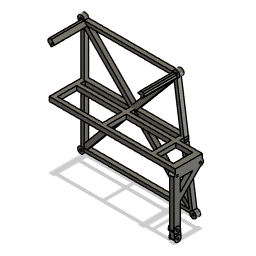
ITX_1 (Autodesk Fusion 360 design; units mm, degrees)
Autodesk Fusion 360 part; units mm, degrees
note: some values were not read from the file. Set by a fixed rule: which face or edge a step refers to.
sketch "草图1" plane through (0, 0, 0) normal (0, 1, 0) x (1, 0, 0)
  line L0 (0, 0) -> (81.5, 0)
  line L1 (81.5, 0) -> (81.5, -40.5)
  line L2 (81.5, -40.5) -> (0, -40.5)
  line L3 (0, -40.5) -> (0, 0)
  line L4 (81.5, -40.5) -> (-5, -40.5)
  line L5 (-5, -40.5) -> (-5, 5)
  line L6 (-5, 5) -> (81.5, 5)
  line L7 (81.5, 5) -> (81.5, -40.5)
  line L8 (0, 0) -> (86.5, 0)
  line L9 (86.5, 0) -> (86.5, -45.5)
  line L10 (86.5, -45.5) -> (0, -45.5)
  line L11 (0, -45.5) -> (0, 0)
  line L12 (-5, 5) -> (86.5, 5)
  line L13 (86.5, 5) -> (86.5, -45.5)
  line L14 (86.5, -45.5) -> (-5, -45.5)
  line L15 (-5, -45.5) -> (-5, 5)
  line L16 (-6, 6) -> (87.5, 6)
  line L17 (87.5, 6) -> (87.5, -46.5)
  line L18 (87.5, -46.5) -> (-6, -46.5)
  line L19 (-6, -46.5) -> (-6, 6)
  line L20 (-1, -41.5) -> (82.5, -41.5)
  line L21 (82.5, -41.5) -> (82.5, 1)
  line L22 (82.5, 1) -> (-1, 1)
  line L23 (-1, 1) -> (-1, -41.5)
  dimension "d1" = 81.5
  dimension "d2" = 40.5
  dimension "d3" = 5
  dimension "d4" = 5
  dimension "d5" = 5
  dimension "d6" = 5
  dimension "d7" = 1
  dimension "d8" = 1
  dimension "d9" = 1
  dimension "d10" = 1
  dimension "d11" = 1
  dimension "d12" = 1
  dimension "d13" = 1
  dimension "d14" = 1
  dimension "d15" = 4
  constraint horizontal L0
  constraint vertical L1
  constraint horizontal L2
  constraint vertical L3
  constraint coincident L0.start L3.end
  constraint horizontal L4
  constraint vertical L5
  constraint horizontal L6
  constraint vertical L7
  constraint horizontal L8
  constraint vertical L9
  constraint horizontal L10
  constraint vertical L11
  constraint horizontal L12
  constraint vertical L13
  constraint horizontal L14
  constraint vertical L15
  constraint horizontal L16
  constraint vertical L17
  constraint horizontal L18
  constraint vertical L19
  constraint horizontal L20
  constraint vertical L21
  constraint horizontal L22
  constraint vertical L23
  measures "d1" distance of L0.start L0.end
  measures "d2" distance of L0.start L2.end
  measures "d3" distance of L3 L5
  measures "d4" distance of L0 L6
  measures "d5" distance of L1 L9
  measures "d6" distance of L4 L10
  measures "d7" distance of L12 L16
  measures "d8" distance of L5 L19
  measures "d9" distance of L10 L18
  measures "d10" distance of L9 L17
  measures "d11" distance of L8 L22
  measures "d12" distance of L3 L23
  measures "d13" distance of L2 L20
  measures "d14" distance of L7 L21
  measures "d15" distance of L9 L21
extrude "拉伸1" add sketch "草图1" along normal blind 160 contours L4 L5 L6 L7 L12 L15 L22 L23 | L7 L8 L12 L13 L21 L22 | L8 L9 L10 L11 L13 L14 L20 L21 | L4 L11 L14 L15 L20 L23 makes body 1
extrude "拉伸2" add sketch "草图1" against normal blind 4 separate body contours L4 L5 L6 L7 L12 L15 L22 L23 | L7 L8 L12 L13 L21 L22 | L8 L9 L10 L11 L13 L14 L20 L21 | L4 L11 L14 L15 L20 L23 makes body 2
extrude "拉伸3" add 2 faces at (54, -1.3333, -1) (82.1667, -1.3333, -1) along direction (0, 0, 1) blind 42.5 separate body on bodies 2 makes body 3
sketch "草图2" plane through (0, 0, -5) normal (0, 0, -1) x (-1, 0, 0)
  line L0 (-86.5, 0) -> (5, 0)
  line L1 (5, 0) -> (5, 160)
  line L2 (5, 160) -> (-86.5, 160)
  line L3 (-86.5, 160) -> (-86.5, 0)
  line L4 (5, 160) -> (-165, 160)
  line L5 (-165, 160) -> (-165, -10)
  line L6 (-165, -10) -> (5, -10)
  line L7 (5, -10) -> (5, 160)
  line L8 (5, 160) -> (-166, 160)
  line L9 (-166, 160) -> (-166, -11)
  line L10 (-166, -11) -> (5, -11)
  line L11 (5, -11) -> (5, 160)
  line L12 (-166, -11) -> (6, -11)
  line L13 (6, -11) -> (6, 161)
  line L14 (6, 161) -> (-166, 161)
  line L15 (-166, 161) -> (-166, -11)
  circle A0 centre (-131.98, 153.83) radius 1.5
  circle A1 centre (0.1, 153.83) radius 1.5
  circle A2 centre (-154.84, -3.65) radius 1.5
  circle A3 centre (0.1, -3.65) radius 1.5
  line L16 (-131.98, 153.83) -> (0.1, 153.83)
  line L17 (-154.84, -3.65) -> (0.1, -3.65)
  circle A4 centre (-131.98, 153.83) radius 4.5
  circle A5 centre (0.1, 153.83) radius 4.5
  circle A6 centre (0.1, -3.65) radius 4.5
  circle A7 centre (-154.84, -3.65) radius 4.5
  line L18 (-131.98, 153.83) -> (-154.84, -3.65)
  line L19 (0.1, 153.83) -> (0.1, -3.65)
  line L20 (-127.48, 153.83) -> (-150.34, -3.65)
  line L21 (-4.4, 153.83) -> (-4.4, -3.65)
  line L22 (0.1, 153.83) -> (4.6, 153.83)
  line L23 (0.1, -3.65) -> (4.6, -3.65)
  line L24 (4.6, -3.65) -> (4.6, 153.83)
  line L25 (-132.6265, 149.3767) -> (-131.3335, 158.2833)
  line L26 (-131.3335, 158.2833) -> (0.0984, 158.33)
  line L27 (-154.1935, 0.8033) -> (-155.4865, -8.1033)
  line L28 (-155.4865, -8.1033) -> (0.0986, -8.15)
  line L29 (-154.1935, 0.8033) -> (0.1, 0.85)
  line L30 (-132.6265, 149.3767) -> (0.1, 149.33)
  line L31 (-132.6265, 149.3767) -> (-4.4, -3.65)
  line L32 (0.1, 0.85) -> (-127.48, 153.83)
  line L33 (-154.1935, 0.8033) -> (-4.4, 153.83)
  line L34 (0.1, 149.33) -> (-150.34, -3.65)
  line L35 (-165, 160) -> (-165, 1)
  dimension "d22" = 170
  dimension "d23" = 170
  dimension "d24" = 1
  dimension "d25" = 1
  dimension "d26" = 1
  dimension "d27" = 1
  dimension "d28" = 3
  dimension "d29" = 3
  dimension "d30" = 3
  dimension "d31" = 3
  dimension "d32" = 132.08
  dimension "d33" = 157.48
  dimension "d34" = 157.48
  dimension "d35" = 154.94
  dimension "d36" = 6.35
  dimension "d37" = 22.86
  dimension "d38" = 10.16
  dimension "d39" = 9
  dimension "d40" = 9
  dimension "d41" = 9
  dimension "d42" = 9
  dimension "d84" = 159
  constraint horizontal L4
  constraint vertical L5
  constraint horizontal L6
  constraint vertical L7
  constraint coincident L1.end L2.start
  constraint horizontal L8
  constraint vertical L9
  constraint horizontal L10
  constraint vertical L11
  constraint horizontal L12
  constraint vertical L13
  constraint horizontal L14
  constraint vertical L15
  constraint coincident A0.centre L16.start
  constraint coincident A1.centre L16.end
  constraint coincident A2.centre L17.start
  constraint coincident A3.centre L17.end
  constraint concentric A2 A7
  constraint coincident A4 L20.start
  constraint coincident L16 L20.start
  constraint coincident A7 L20.end
  constraint coincident L17 L20.end
  constraint coincident A5 L21.start
  constraint coincident L16 L21.start
  constraint coincident L17 L21.end
  constraint coincident A6 L21.end
  constraint tangent A6 L21
  constraint coincident A5 L22.end
  constraint perpendicular L7 L22
  constraint coincident A6 L23.end
  constraint perpendicular L7 L23
  constraint coincident A4 L25.start
  constraint coincident L18 L25.start
  constraint coincident A4 L25.end
  constraint parallel L18 L25
  constraint coincident A5 L26.end
  constraint tangent A5 L26
  constraint coincident A7 L27.start
  constraint coincident L18 L27.start
  constraint coincident A7 L27.end
  constraint parallel L18 L27
  constraint coincident A6 L28.end
  constraint tangent A6 L28
  constraint coincident A6 L29.end
  constraint coincident L19 L29.end
  constraint coincident A5 L30.end
  constraint coincident L19 L30.end
  constraint perpendicular L4 L35
  measures "d22" distance of L1.end L4.end
  measures "d23" distance of L1.end L6.end
  measures "d24" distance of L5 L9
  measures "d25" distance of L6 L10
  measures "d26" distance of L4 L14
  measures "d27" distance of L11 L13
  measures "d28" diameter of A0
  measures "d29" diameter of A1
  measures "d30" diameter of A2
  measures "d31" diameter of A3
  measures "d32" horizontal distance of A0.centre A1.centre
  measures "d33" vertical distance of A0.centre A2.centre
  measures "d34" vertical distance of A1.centre A3.centre
  measures "d35" horizontal distance of A2.centre A3.centre
  measures "d36" distance of L6 A2.centre
  measures "d37" horizontal distance of A0.centre A2.centre
  measures "d38" distance of L5 A2.centre
  measures "d39" diameter of A4
  measures "d40" diameter of A5
  measures "d41" diameter of A6
  measures "d42" diameter of A7
  measures "d84" distance of L4.end L35.end
extrude "拉伸4" add sketch "草图2" along normal blind 6 separate body contours L0 A6 L19 | L0 A3 L17 A6 L19 | A3 L17 A6 L23 | L0 A6 L19 | A2 L17 A7 L27 L28 | A2 L17 A7 L18 L27 | L0 A3 A6 L19 L23 | A2 A7 L18 L27 | A7 L28 | A1 A5 L19 L22 | A1 L16 A5 L19 | A4 L30 | A0 A4 L18 L25 | A0 L16 A4 L18 L20 L25 L30 | A1 L16 A5 L22 | A0 L16 A4 L25 | A4 L20 makes body 4 at (-4.2466, 152.082, -9) makes body 5 at (-4.5776, -4.0981, -7) makes body 6 at (127.4856, 154.0543, -7) makes body 7 at (150.3624, -3.2019, -9)
extrude "拉伸5" add sketch "草图2" along normal blind 6 separate body contours L0 L3 L29 L31 | L0 L3 L17 L29 L31 L34 | L0 L21 L29 L31 | L0 L21 L31 | L21 L29 L32 | L19 L21 L32 L34 | L0 A6 L21 L29 | L0 A6 L21 | L20 L29 L34 | A7 L20 L29 | L20 L29 L33 | L18 L20 L31 L33 | A5 L21 L30 | L21 L30 L34 | A4 L20 L30 L31 | L3 L16 L30 L33 | L21 L30 L33 | A4 L20 L30 | L3 L16 L30 L32 | A4 L20 L30 L32 makes body 8
extrude "拉伸6" add sketch "草图2" along normal blind 6 separate body contours L21 L29 L31 L32 L34 | L3 L20 L29 L33 L34 | L3 L31 L33 L34 | L31 L32 L33 L34 | L3 L31 L32 L33 | L21 L30 L32 L33 L34 | L3 L20 L30 L31 L32 makes body 9
move_body "移动1" bodies 1 3 2 to x (1, 0, 0) y (0, 1, 0) z (0, 0, 1) at (10, 0, 0)
move_body "移动2" bodies 1 3 2 to x (0, 1, 0) y (-1, 0, 0) z (0, 0, 1) at (92.5, -100.5, 0)
move_body "移动3" bodies 2 3 1 to x (1, 0, 0) y (0, 1, 0) z (0, 0, 1) at (69.5, 84.5, 0)
sketch "草图3" plane through (166, 0, 0) normal (1, 0, 0) x (0, 0, -1)
  line L0 (1, -7) -> (1, 76.5)
  line L1 (1, 76.5) -> (-41.5, 76.5)
  line L2 (-41.5, 76.5) -> (-41.5, -7)
  line L3 (-41.5, -7) -> (1, -7)
  circle A0 centre (-36, 73) radius 1.5
  circle A1 centre (-4, 73.0152) radius 1.5
  circle A2 centre (-35, -2.6) radius 1.5
  circle A3 centre (-36, 8.2) radius 1.5
  line L4 (-36, 8.2) -> (-36, 73)
  circle A4 centre (-35, -2.6) radius 4.4
  circle A5 centre (-36, 8.2) radius 4.4
  circle A6 centre (-36, 73) radius 4.4
  circle A7 centre (-4, 73.0152) radius 4.4
  line L5 (-33.3335, 76.5) -> (-6.6863, 76.5)
  line L6 (-36, 68.6) -> (-3.9979, 68.6152)
  line L7 (-36, 73) -> (-40.4, 73)
  line L8 (-36, 8.2) -> (-40.4, 8.2)
  line L9 (-35, -2.6) -> (-39.4, -2.6)
  line L10 (-39.4, -2.6) -> (-40.4, 8.2)
  line L11 (-40.4, 8.2) -> (-40.4, 73)
  line L12 (-36, 8.2) -> (-31.6, 8.2)
  line L13 (-31.6, 8.2) -> (-31.6, 73)
  line L14 (-36, 73) -> (-31.6, 73)
  line L15 (-35, -2.6) -> (-30.6, -2.6)
  line L16 (-31.6, 8.2) -> (-30.6, -2.6)
  line L17 (-4, 73.0152) -> (0.4, 73.0152)
  line L18 (-3.9979, 68.6152) -> (-31.6, 40.6)
  line L19 (-6.6863, 76.5) -> (-31.6, 51.2134)
  dimension "d50" = 3
  dimension "d51" = 3
  dimension "d52" = 3
  dimension "d53" = 3
  dimension "d54" = 32
  dimension "d56" = 15.2
  dimension "d57" = 4.4
  dimension "d58" = 36
  dimension "d59" = 37
  dimension "d60" = 8.8
  dimension "d61" = 8.8
  dimension "d62" = 8.8
  dimension "d63" = 8.8
  constraint coincident A3.centre L4.start
  constraint coincident A0.centre L4.end
  constraint concentric A2 A4
  constraint concentric A3 A5
  constraint concentric A0 A6
  constraint concentric A1 A7
  constraint coincident A6 L5.start
  constraint coincident L1 L5.start
  constraint coincident A7 L5.end
  constraint coincident L1 L5.end
  constraint coincident A6 L6.start
  constraint coincident L4 L6.start
  constraint coincident A7 L6.end
  constraint tangent A7 L6
  constraint coincident A6 L7.end
  constraint perpendicular L4 L7
  constraint coincident A5 L8.end
  constraint perpendicular L4 L8
  constraint coincident A2.centre A4.centre
  constraint coincident A4 L9.end
  constraint parallel L8 L9
  constraint coincident A5 L12.end
  constraint parallel L8 L12
  constraint coincident A6 L13.end
  constraint tangent A6 L13
  constraint coincident A4 L15.end
  constraint parallel L9 L15
  constraint coincident A1.centre A7.centre
  constraint coincident A7 L17.end
  constraint perpendicular L0 L17
  constraint midpoint L13 L18.end
  constraint coincident L13 L19.end
  constraint parallel L18 L19
  measures "d50" diameter of A0
  measures "d51" diameter of A1
  measures "d52" diameter of A2
  measures "d53" diameter of A3
  measures "d54" distance of A0.centre A1.centre
  measures "d56" distance of L3 A3.centre
  measures "d57" distance of L3 A2.centre
  measures "d58" distance of L0 A2.centre
  measures "d59" distance of L0 A3.centre
  measures "d60" diameter of A4
  measures "d61" diameter of A5
  measures "d62" diameter of A6
  measures "d63" diameter of A7
extrude "拉伸7" add sketch "草图3" along normal blind 8 separate body contours A2 A4 L9 L15 | L1 A7 L19 | A2 A4 L9 L15 L16 | A4 L16 | A7 L19 | A3 A5 L8 L10 L12 | A5 L10 | L1 A0 A6 L7 L14 | A3 L4 A5 L12 | A3 L4 A5 L8 | A0 L4 A6 L14 | A0 L4 A6 L7 makes body 10 at (171.3333, 72.3225, 40.3475) makes body 11 at (168.6667, -3.0381, 30.6219) makes body 12 at (171.3333, 76.2221, 7.0126) makes body 13 at (168.6667, 7.7619, 31.6219)
extrude "拉伸8" add sketch "草图3" along normal blind 8 separate body contours A4 A5 L10 L16 | L1 A6 A7 L5 L6 L13 L19 | A7 L6 L19 | L6 L13 L18 L19 | L4 A5 L6 L13 | L4 A5 A6 L11 | A6 L6 L13 makes body 14
extrude "拉伸9" add 3 faces at (168.6667, 76.5, 35.1112) (168.6667, 76.5, 15.5687) (171.3333, 76.5, 3.1046) along direction (0, 1, 0) blind 6 separate body on bodies 10 12 14 makes body 15
extrude "拉伸10" add 3 faces at (166, 80.5, 35.1112) (166, 78.5, 15.5687) (166, 78.5, 3.1046) along direction (-1, 0, 0) blind 166.1 on bodies 15 bodies 14 15 10 12
extrude "拉伸11" add 1 faces at (113.3, 80.5, 1.3137) along direction (0, 0, -1) blind 12.314 separate body on bodies 14 makes body 16
extrude "拉伸12" cut 1 faces at (174, 78.5, -2.791) along direction (-1, 0, 0) blind 31.173 on bodies 16 bodies 8 16
combine "合并1" operation add target body 14 tool bodies 16
sketch "草图4" plane through (0, 82.5, 0) normal (0, 1, 0) x (-1, 0, 0)
  line L0 (0.1, 38.6665) -> (-174, 38.6665)
  line L1 (-174, 38.6665) -> (-174, 1.3137)
  line L2 (-174, 1.3137) -> (-142.827, 1.3137)
  line L3 (-142.827, 1.3137) -> (-142.827, -11.0003)
  line L4 (-142.827, -11.0003) -> (0.1, -11.0003)
  line L5 (0.1, -11.0003) -> (0.1, 38.6665)
  line L6 (0.1, 38.6665) -> (-5.9, 38.6665)
  line L7 (-174, 38.6665) -> (-166, 38.6665)
  line L8 (-142.827, 1.3137) -> (-142.827, 38.6665)
  line L9 (-142.827, 38.6665) -> (-136.827, 38.6665)
  line L10 (-71.3635, -11.0003) -> (-71.3635, 38.6665)
  line L11 (-71.3635, 38.6665) -> (-68.3635, 38.6665)
  line L12 (-71.3635, 38.6665) -> (-74.3635, 38.6665)
  line L13 (-5.9, 38.6665) -> (-68.3635, 38.6665)
  line L14 (-68.3635, 38.6665) -> (-68.3635, -11.0003)
  line L15 (-68.3635, -11.0003) -> (-5.9, -11.0003)
  line L16 (-5.9, -11.0003) -> (-5.9, 38.6665)
  line L17 (-74.3635, 38.6665) -> (-136.827, 38.6665)
  line L18 (-136.827, 38.6665) -> (-136.827, -11.0003)
  line L19 (-136.827, -11.0003) -> (-74.3635, -11.0003)
  line L20 (-74.3635, -11.0003) -> (-74.3635, 38.6665)
  line L21 (-5.9, 38.6665) -> (-142.827, 38.6665)
  line L22 (-142.827, 38.6665) -> (-142.827, -4.8433)
  line L23 (-142.827, -4.8433) -> (-5.9, -4.8433)
  line L24 (-5.9, -4.8433) -> (-5.9, 38.6665)
  line L25 (0.1, 38.6665) -> (-172, 38.6665)
  line L26 (-172, 38.6665) -> (-172, 33.3335)
  line L27 (-172, 33.3335) -> (0.1, 33.3335)
  line L28 (0.1, 33.3335) -> (0.1, 38.6665)
  line L29 (-174, 6.6863) -> (-142.827, 6.6863)
  line L30 (-142.827, 6.6863) -> (-142.827, 1.3137)
  line L31 (-142.827, 1.3137) -> (-174, 1.3137)
  line L32 (-174, 1.3137) -> (-174, 6.6863)
  line L33 (-142.827, 1.3137) -> (0.1, 1.3137)
  line L34 (0.1, 1.3137) -> (0.1, 6.6863)
  line L35 (0.1, 6.6863) -> (-142.827, 6.6863)
  line L36 (-142.827, 6.6863) -> (-142.827, 1.3137)
  line L37 (-172, 33.3335) -> (-166, 33.3335)
  line L38 (-166, 33.3335) -> (-166, 38.6665)
  line L39 (-166, 38.6665) -> (-172, 38.6665)
  line L40 (-172, 38.6665) -> (-172, 33.3335)
  line L41 (-166, 33.3335) -> (-172, 33.3335)
  line L42 (-172, 33.3335) -> (-172, 1.3137)
  line L43 (-172, 1.3137) -> (-166, 1.3137)
  line L44 (-166, 1.3137) -> (-166, 33.3335)
  dimension "d76" = 6
  dimension "d77" = 6
  dimension "d78" = 3
  dimension "d79" = 3
  constraint coincident L0.start L5.end
  constraint perpendicular L5 L6
  constraint coincident L0.end L1.start
  constraint coincident L0 L7.end
  constraint perpendicular L1 L7
  constraint coincident L2.end L3.start
  constraint coincident L0 L8.end
  constraint perpendicular L0 L8
  constraint perpendicular L8 L9
  constraint midpoint L4 L10.start
  constraint coincident L0 L10.end
  constraint perpendicular L0 L10
  constraint perpendicular L10 L11
  constraint perpendicular L10 L12
  constraint horizontal L13
  constraint vertical L14
  constraint horizontal L15
  constraint vertical L16
  constraint coincident L4 L14.end
  constraint horizontal L17
  constraint vertical L18
  constraint horizontal L19
  constraint vertical L20
  constraint coincident L4 L18.end
  constraint horizontal L21
  constraint vertical L22
  constraint horizontal L23
  constraint vertical L24
  constraint midpoint L3 L22.end
  constraint horizontal L25
  constraint vertical L26
  constraint horizontal L27
  constraint vertical L28
  constraint horizontal L29
  constraint vertical L30
  constraint horizontal L31
  constraint vertical L32
  constraint coincident L2.end L29.start
  constraint horizontal L33
  constraint vertical L34
  constraint horizontal L35
  constraint vertical L36
  constraint coincident L5 L34.end
  constraint horizontal L37
  constraint vertical L38
  constraint horizontal L39
  constraint vertical L40
  constraint horizontal L41
  constraint vertical L42
  constraint horizontal L43
  constraint vertical L44
  constraint coincident L31 L42.end
  measures "d76" distance of L0.start L6.end
  measures "d77" distance of L8.end L9.end
  measures "d78" distance of L10.end L11.end
  measures "d79" distance of L10.end L12.end
extrude "拉伸13" cut sketch "草图4" against normal blind 6 contours L14 L16 L24 L27 L35 | L14 L16 L23 L24 L33 | L18 L20 L27 L35 | L8 L22 L27 L29 L44 | L18 L20 L23 L33 bodies 14
extrude "拉伸14" cut sketch "草图3" along normal blind 2 contours A4 A5 L10 L16 | L1 A6 A7 L5 L6 L13 L19 | A7 L6 L19 | L6 L13 L18 L19 | L4 A5 L6 L13 | L4 A5 A6 L11 | A6 L6 L13 bodies 14
extrude "拉伸15" add sketch "草图2" against normal blind 45.4 separate body contours A5 L21 L30 | A1 L16 A5 L19 | L21 L30 L34 | A0 L16 A4 L18 L20 L25 L30 | A4 L20 L30 L31 | L21 L30 L33 | A4 L20 L30 | A4 L20 L30 L32 makes body 17 at (1.4, 147.8047, 10.1333) makes body 18 at (131.3479, 147.8509, 10.1333)
hidden bodies 1 2 3
